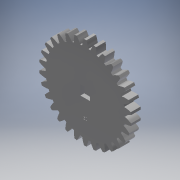
# Autodesk Inventor part: 30_teeth
Saved by Autodesk Inventor 2019 (Build 230136000, 136)
## iProperties
Created: 2020-02-24
Part Number: 30_teeth
Material: Steel
Document SubType Name: Modeling
Designer: Jeff
Categories: <?xml version="1.0" encoding="UTF-16"?> <MemberInstance><Categories><FamilyTemplate><FamilyTemplateParameter ValueType="xs:double" Id="1" ObjectReferenceKey="da_z" ObjectType="kUserParameterObject"/><FamilyTemplateParameter ValueType="xs:double" Id="2" ObjectReferenceKey="da_b" ObjectType="kUserParameterObject"/><FamilyTemplateParameter ValueType="xs:double" Id="3" ObjectReferenceKey="da_beta" ObjectType="kUserParameterObject"/><FamilyTemplateParameter ValueType="xs:double" Id="4" ObjectReferenceKey="da_da" ObjectType="kUserParameterObject"/><FamilyTemplateParameter ValueType="xs:double" Id="5" ObjectReferenceKey="da_aw" ObjectType="kUserParameterObject"/><FamilyTemplateParameter ValueType="xs:string" Id="6" ObjectReferenceKey="EAIAABAAAACIAQAAAAAAAIAAAAAAAAAA" ObjectType="83910656" SubObjectId="SurfaceGeometry"/></FamilyTemplate><ParamToTemplateMap><ParamToTemplate CategoryParameter="//CategoryParameter[@InternalName='046C89C9-8512-4d59-83FE-43B91F4F132A']" TemplateParameter="1"/><ParamToTemplate CategoryParameter="//CategoryParameter[@InternalName='2552DF32-E462-4b46-AEBF-C6C7768E72AC']" TemplateParameter="2"/><ParamToTemplate CategoryParameter="//CategoryParameter[@InternalName='C9EE641D-15FC-4fae-A226-E94C4372FDD7']" TemplateParameter="3"/><ParamToTemplate><ParamToTemplate CategoryParameter="//CategoryParameter[@InternalName='00B6519A-459B-49c7-AD84-2E56D39A5744']" ConstantValue="0.000000"/></ParamToTemplate><ParamToTemplate><ParamToTemplate CategoryParameter="//CategoryParameter[@InternalName='04B31F0E-C7A6-4894-AA32-9629BEFACF47']" ConstantValue="1.000000"/></ParamToTemplate><ParamToTemplate><ParamToTemplate CategoryParameter="//CategoryParameter[@InternalName='43CBEC2E-7847-49e7-A936-2F7889FCB2D9']" ConstantValue="0.250000"/></ParamToTemplate><ParamToTemplate><ParamToTemplate CategoryParameter="//CategoryParameter[@InternalName='B1EFC894-105D-4ebd-86BF-FA20ED196853']" ConstantValue="0.350000"/></ParamToTemplate><ParamToTemplate><ParamToTemplate CategoryParameter="//CategoryParameter[@InternalName='51175063-3D10-4879-93E8-6246FE8B403D']" ConstantValue="2060000000.000000"/></ParamToTemplate><ParamToTemplate><ParamToTemplate CategoryParameter="//CategoryParameter[@InternalName='A3A52E27-4454-46a9-B0BD-C932399B70AF']" ConstantValue="0.300000"/></ParamToTemplate><ParamToTemplate><ParamToTemplate CategoryParameter="//CategoryParameter[@InternalName='91B76062-C214-41d9-B1B9-14D2AB99603D']" ConstantValue="0.300000"/></ParamToTemplate><ParamToTemplate><ParamToTemplate CategoryParameter="//CategoryParameter[@InternalName='374E806E-8B8A-4dda-A9AA-1039D6500AD2']" ConstantValue="3.333333"/></ParamToTemplate><ParamToTemplate><ParamToTemplate CategoryParameter="//CategoryParameter[@InternalName='2D373A89-B862-43d6-8D0B-0CBF12AB9F6C']" ConstantValue="0.349066"/></ParamToTemplate><ParamToTemplate CategoryParameter="//CategoryParameter[@InternalName='37777632-D6A2-4fac-9D53-DB8ACD95C989']" TemplateParameter="4"/><ParamToTemplate CategoryParameter="//CategoryParameter[@InternalName='FD1017F1-B727-4f7e-9707-0F86F1FF9423']" TemplateParameter="5"/><ParamToTemplate><ParamToTemplate CategoryParameter="//CategoryParameter[@InternalName='9E1B4470-B2D3-4ff1-B813-535BB4CDF51A']" ConstantValue="3520000.000000"/></ParamToTemplate><ParamToTemplate><ParamToTemplate CategoryParameter="//CategoryParameter[@InternalName='F8452263-BFF6-458c-9FB1-07C4B99E95CD']" ConstantValue="11400000.000000"/></ParamToTemplate><ParamToTemplate><ParamToTemplate CategoryParameter="//CategoryParameter[@InternalName='3E3BB259-FD49-497f-8171-6EBC954A3479']" ConstantValue="2.000000"/></ParamToTemplate><ParamToTemplate CategoryParameter="//CategoryParameter[@InternalName='27C3BAF2-7550-4e4b-AE2C-0DB134B7D9B7']" TemplateParameter="6"/></ParamToTemplateMap><Category DisplayName="Gear" InternalName="DC85795E-93AB-48d5-8EEE-5A27447B64BD" Mnemonic="Gear"><CategoryParameter DisplayName="z" InternalName="046C89C9-8512-4d59-83FE-43B91F4F132A" Mnemonic="z"/><CategoryParameter DisplayName="b" InternalName="2552DF32-E462-4b46-AEBF-C6C7768E72AC" Mnemonic="b"/><CategoryParameter DisplayName="||b|" InternalName="C9EE641D-15FC-4fae-A226-E94C4372FDD7" Mnemonic="beta"/><CategoryParameter DisplayName="x" InternalName="00B6519A-459B-49c7-AD84-2E56D39A5744" Mnemonic="x"/><CategoryParameter DisplayName="a*" InternalName="04B31F0E-C7A6-4894-AA32-9629BEFACF47" Mnemonic="a"/><CategoryParameter DisplayName="c*" InternalName="43CBEC2E-7847-49e7-A936-2F7889FCB2D9" Mnemonic="c"/><CategoryParameter DisplayName="r|.f|*" InternalName="B1EFC894-105D-4ebd-86BF-FA20ED196853" Mnemonic="rf"/><CategoryParameter DisplayName="E" InternalName="51175063-3D10-4879-93E8-6246FE8B403D" Mnemonic="E"/><CategoryParameter DisplayName="||m|" InternalName="A3A52E27-4454-46a9-B0BD-C932399B70AF" Mnemonic="mi"/><Category DisplayName="SpurGear" InternalName="26C5A22E-A91E-4dfd-A3B3-23CCAFAE1764" Mnemonic="SpurGear"><CategoryParameter DisplayName="m" InternalName="91B76062-C214-41d9-B1B9-14D2AB99603D" Mnemonic="m"/><CategoryParameter DisplayName="P" InternalName="374E806E-8B8A-4dda-A9AA-1039D6500AD2" Mnemonic="PP"/><CategoryParameter DisplayName="||a|" InternalName="2D373A89-B862-43d6-8D0B-0CBF12AB9F6C" Mnemonic="alpha"/><CategoryParameter DisplayName="d|.a|" InternalName="37777632-D6A2-4fac-9D53-DB8ACD95C989" Mnemonic="da"/><CategoryParameter DisplayName="a|.w|" InternalName="FD1017F1-B727-4f7e-9707-0F86F1FF9423" Mnemonic="aw"/><CategoryParameter DisplayName="||s||.Flim|" InternalName="9E1B4470-B2D3-4ff1-B813-535BB4CDF51A" Mnemonic="sFlim"/><CategoryParameter DisplayName="||s||.Hlim|" InternalName="F8452263-BFF6-458c-9FB1-07C4B99E95CD" Mnemonic="sHlim"/><CategoryParameter DisplayName="type" InternalName="3E3BB259-FD49-497f-8171-6EBC954A3479" Mnemonic="type"/><CategoryParameter DisplayName="PitchDiameter" InternalName="27C3BAF2-7550-4e4b-AE2C-0DB134B7D9B7" Mnemonic="IDS_PITCHDIAM"/></Category></Category></Categories></MemberInstance>
Density: 1 g/cm^3
Appearance: Steel
CustomPartVersion: 1
Author: Jeff
Autodesk Inventor part; units mm, degrees
sketch "Sketch1" plane through (0, 0, 0) normal (0, 0, 1) x (1, 0, 0)
  circle A0 centre (0, 0) radius 48
  dimension "d0" = 96
  constraints: 1 centre point
  measures "d0" diameter of A0
extrude "Extrusion1" add sketch "Sketch1" along normal blind 10
ref_plane "Work Plane2" through (0, 0, 5) normal (0, 0, 1) x (1, 0, 0)
sketch "Sketch2" plane through (0, 0, 0) normal (0, 0, -1) x (-1, 0, 0)
  circle A0 centre (0, 0) radius 48 projected
  circle A1 centre (0, 0) radius 45
  dimension "d3" = 90
  constraints: 1 centre point, 1 coincident
  measures "d3" diameter of A1
surface extrude "Pitch Diameter" sketch "Sketch2" against normal through all shown no curves A1
ref_plane "Work Plane8" through (0, 0, 0) normal (0.9945219, 0.1045285, 0) x (0, 0, 1)
ref_plane "Work Plane9" through (0, 0, 0) normal (1, 0, 0) x (0, 1, 0)
spur gear teeth "Spur Gear" teeth 30 pitch diameter 90 tip diameter 96 root diameter 82.5 face width 10 start plane through (0, 0, 0) normal (0, 0, -1) x (-1, 0, 0)
sketch "Sketch3" plane through (0, 0, 10) normal (0, 0, 1) x (1, 0, 0)
  line L0 (-5, 5) -> (5, 5)
  line L1 (5, 5) -> (5, -5)
  line L2 (5, -5) -> (-5, -5)
  line L3 (-5, -5) -> (-5, 5)
  line L4 (-5, -28.0614) -> (-5, -18.0614) construction
  line L5 (-5, -18.0614) -> (5, -18.0614) construction
  line L6 (5, -18.0614) -> (5, -28.0614) construction
  line L7 (5, -28.0614) -> (-5, -28.0614) construction
  arc A0 (-3.2364, -41.1228) -> (-1.2565, -47.9836) centre (26.3871, -36.2898) ccw projected
  line L8 (-3.2364, -41.1228) -> (-3.2364, -5)
  spline S0 degree 2 poles (-1.2229, -21.8459) (-1.3323, -21.8459) (-1.5486, -21.8993) (-1.6532, -21.9407) knots 0 0 0 1 2 2 2
  spline S1 degree 2 poles (-1.6532, -21.9407) (-1.7504, -21.982) (-1.8938, -22.0695) (-1.9498, -22.1084) knots 0 0 0 1 2 2 2
  line L9 (-1.9498, -22.1084) -> (-1.9741, -22.1084)
  line L10 (-1.9741, -22.1084) -> (-1.9741, -21.683)
  spline S2 degree 2 poles (-1.9741, -21.683) (-1.8428, -21.6125) (-1.393, -21.4982) (-1.1912, -21.4982) knots 0 0 0 1 2 2 2
  spline S3 degree 2 poles (-1.1912, -21.4982) (-0.987, -21.4982) (-0.6831, -21.5809) (-0.5592, -21.6684) knots 0 0 0 1 2 2 2
  spline S4 degree 2 poles (-0.5592, -21.6684) (-0.4279, -21.7632) (-0.2917, -22.0379) (-0.2917, -22.2227) knots 0 0 0 1 2 2 2
  spline S5 degree 2 poles (-0.2917, -22.2227) (-0.2917, -22.4707) (-0.6175, -22.8451) (-0.846, -22.8937) knots 0 0 0 1 2 2 2
  line L11 (-0.846, -22.8937) -> (-0.846, -22.9228)
  spline S6 degree 2 poles (-0.846, -22.9228) (-0.7512, -22.9423) (-0.5348, -23.0298) (-0.4425, -23.1173) knots 0 0 0 1 2 2 2
  spline S7 degree 2 poles (-0.4425, -23.1173) (-0.3501, -23.2024) (-0.2334, -23.4747) (-0.2334, -23.6716) knots 0 0 0 1 2 2 2
  spline S8 degree 2 poles (-0.2334, -23.6716) (-0.2334, -23.8734) (-0.372, -24.2162) (-0.4984, -24.3475) knots 0 0 0 1 2 2 2
  spline S9 degree 2 poles (-0.4984, -24.3475) (-0.6297, -24.4836) (-1.0016, -24.6246) (-1.2374, -24.6246) knots 0 0 0 1 2 2 2
  spline S10 degree 2 poles (-1.2374, -24.6246) (-1.4635, -24.6246) (-1.906, -24.5152) (-2.0567, -24.4399) knots 0 0 0 1 2 2 2
  line L12 (-2.0567, -24.4399) -> (-2.0567, -24.0144)
  line L13 (-2.0567, -24.0144) -> (-2.0276, -24.0144)
  spline S11 degree 2 poles (-2.0276, -24.0144) (-1.9011, -24.1068) (-1.4733, -24.277) (-1.2618, -24.277) knots 0 0 0 1 2 2 2
  spline S12 degree 2 poles (-1.2618, -24.277) (-1.1378, -24.277) (-0.8898, -24.1992) (-0.8071, -24.1092) knots 0 0 0 1 2 2 2
  spline S13 degree 2 poles (-0.8071, -24.1092) (-0.7269, -24.0193) (-0.6418, -23.8053) (-0.6418, -23.6425) knots 0 0 0 1 2 2 2
  spline S14 degree 2 poles (-0.6418, -23.6425) (-0.6418, -23.4796) (-0.7366, -23.2681) (-0.8217, -23.2073) knots 0 0 0 1 2 2 2
  spline S15 degree 2 poles (-0.8217, -23.2073) (-0.9068, -23.1465) (-1.1378, -23.1003) (-1.2739, -23.1003) knots 0 0 0 1 2 2 2
  line L14 (-1.2739, -23.1003) -> (-1.4441, -23.1003)
  line L15 (-1.4441, -23.1003) -> (-1.4441, -22.7673)
  line L16 (-1.4441, -22.7673) -> (-1.3104, -22.7673)
  spline S16 degree 2 poles (-1.3104, -22.7673) (-1.0405, -22.7673) (-0.7002, -22.5096) (-0.7002, -22.264) knots 0 0 0 1 2 2 2
  spline S17 degree 2 poles (-0.7002, -22.264) (-0.7002, -22.1498) (-0.7877, -21.9869) (-0.8582, -21.9382) knots 0 0 0 1 2 2 2
  spline S18 degree 2 poles (-0.8582, -21.9382) (-0.9335, -21.8872) (-1.1183, -21.8459) (-1.2229, -21.8459) knots 0 0 0 1 2 2 2
  spline S19 degree 2 poles (2.0859, -23.0614) (2.0859, -23.8686) (1.6167, -24.6246) (1.128, -24.6246) knots 0 0 0 1 2 2 2
  spline S20 degree 2 poles (1.128, -24.6246) (0.6321, -24.6246) (0.1677, -23.854) (0.1677, -23.0639) knots 0 0 0 1 2 2 2
  spline S21 degree 2 poles (0.1677, -23.0639) (0.1677, -22.2519) (0.637, -21.5006) (1.128, -21.5006) knots 0 0 0 1 2 2 2
  spline S22 degree 2 poles (1.128, -21.5006) (1.6216, -21.5006) (2.0859, -22.2786) (2.0859, -23.0614) knots 0 0 0 1 2 2 2
  spline S23 degree 2 poles (1.5705, -23.9755) (1.6288, -23.8272) (1.6775, -23.3702) (1.6775, -23.0614) knots 0 0 0 1 2 2 2
  spline S24 degree 2 poles (1.6775, -23.0614) (1.6775, -22.7527) (1.6288, -22.298) (1.5681, -22.1449) knots 0 0 0 1 2 2 2
  spline S25 degree 2 poles (1.5681, -22.1449) (1.5073, -21.9917) (1.2958, -21.8337) (1.128, -21.8337) knots 0 0 0 1 2 2 2
  spline S26 degree 2 poles (1.128, -21.8337) (0.9603, -21.8337) (0.7439, -21.9917) (0.6807, -22.1498) knots 0 0 0 1 2 2 2
  spline S27 degree 2 poles (0.6807, -22.1498) (0.6199, -22.3029) (0.5762, -22.7697) (0.5762, -23.0639) knots 0 0 0 1 2 2 2
  spline S28 degree 2 poles (0.5762, -23.0639) (0.5762, -23.3799) (0.6151, -23.8029) (0.6783, -23.9682) knots 0 0 0 1 2 2 2
  spline S29 degree 2 poles (0.6783, -23.9682) (0.7366, -24.1238) (0.953, -24.2916) (1.128, -24.2916) knots 0 0 0 1 2 2 2
  spline S30 degree 2 poles (1.128, -24.2916) (1.2934, -24.2916) (1.5097, -24.1335) (1.5705, -23.9755) knots 0 0 0 1 2 2 2
  point P0 (0, 0)
  point P1 (0, 5)
  point P2 (5, 0)
  point P3 (0, -18.0614)
  point P4 (-5, -23.0614)
  point P5 (-3.2364, -23.0614)
  dimension "d49" = 10
  dimension "d50" = 10
  dimension "d56" = 10
  dimension "d57" = 10
  constraints: 10 end point, 5 midpoint, 2 horizontal, 2 horizontal alignment, 2 parallel, 2 perpendicular, 1 point on line, 1 vertical alignment, 2 other
  measures "d49" distance of L1.end L2.end
  measures "d50" distance of L0.end L1.end
  measures "d56" distance between parallel lines of L6 L4
  measures "d57" distance between parallel lines of L5 L7
extrude "Extrusion2" cut sketch "Sketch3" against normal blind 4
sketch "Sketch4" plane through (0, 0, 0) normal (0, 0, -1) x (-1, 0, 0)
  circle A0 centre (0, 0) radius 7.5
  dimension "d53" = 15
  constraints: 1 centre point, 1 coincident
  measures "d53" diameter of A0
extrude "Extrusion3" cut sketch "Sketch4" against normal blind 4
equation "\"d0\" = da_da"
equation "\"d1\" = da_b"
equation "\"d3\" = da_dw"
equation "\"da_da\" = 96"
equation "\"da_b\" = 10"
equation "\"da_dw\" = 90"
body "Solid1"
body "Srf1"
